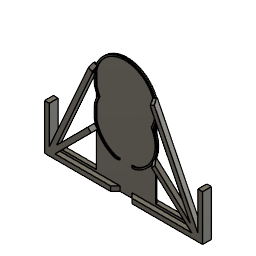
single_jig_wafer_indexer (Autodesk Fusion 360 design; units mm, degrees)
part number: 2026-08-07-17-12-09-687
Autodesk Fusion 360 part; units mm, degrees
(part 1 of 2)
ref_plane "WorkPlane1" through (0, 0, 2) normal (0, 0, 1) x (1, 0, 0)
ref_plane "WorkPlane2" through (0, 0, 3.5) normal (0, 0, 1) x (1, 0, 0)
ref_plane "WorkPlane3" through (0, 0, 10) normal (0, 0, 1) x (1, 0, 0)
ref_plane "WorkPlane4" through (0, 0, 10.2) normal (0, 0, 1) x (1, 0, 0)
ref_plane "WorkPlane5" through (0, 0, -5) normal (0, 0, 1) x (1, 0, 0)
sketch "Front Nest Base Sketch" plane through (0, 0, 0) normal (0, 0, 1) x (1, 0, 0)
  line L0 (174.19, 84.35) -> (174.1396, 86.6618)
  line L1 (174.1396, 86.6618) -> (173.9883, 88.9693)
  line L2 (173.9883, 88.9693) -> (173.7366, 91.2679)
  line L3 (173.7366, 91.2679) -> (173.3848, 93.5534)
  line L4 (173.3848, 93.5534) -> (172.9337, 95.8213)
  line L5 (172.9337, 95.8213) -> (172.3841, 98.0674)
  line L6 (172.3841, 98.0674) -> (171.737, 100.2874)
  line L7 (171.737, 100.2874) -> (170.9937, 102.4771)
  line L8 (170.9937, 102.4771) -> (170.1556, 104.6322)
  line L9 (170.1556, 104.6322) -> (169.2243, 106.7488)
  line L10 (169.2243, 106.7488) -> (168.2016, 108.8227)
  line L11 (168.2016, 108.8227) -> (167.0893, 110.85)
  line L12 (167.0893, 110.85) -> (165.8897, 112.8269)
  line L13 (165.8897, 112.8269) -> (164.6051, 114.7496)
  line L14 (164.6051, 114.7496) -> (163.2377, 116.6144)
  line L15 (163.2377, 116.6144) -> (161.7904, 118.4177)
  line L16 (161.7904, 118.4177) -> (160.2657, 120.1563)
  line L17 (160.2657, 120.1563) -> (158.6667, 121.8267)
  line L18 (158.6667, 121.8267) -> (156.9963, 123.4257)
  line L19 (156.9963, 123.4257) -> (155.2577, 124.9504)
  line L20 (155.2577, 124.9504) -> (153.4544, 126.3977)
  line L21 (153.4544, 126.3977) -> (151.5896, 127.7651)
  line L22 (151.5896, 127.7651) -> (149.6669, 129.0497)
  line L23 (149.6669, 129.0497) -> (147.69, 130.2493)
  line L24 (147.69, 130.2493) -> (145.6627, 131.3616)
  line L25 (145.6627, 131.3616) -> (143.5888, 132.3843)
  line L26 (143.5888, 132.3843) -> (141.4722, 133.3156)
  line L27 (141.4722, 133.3156) -> (139.3171, 134.1537)
  line L28 (139.3171, 134.1537) -> (137.1274, 134.897)
  line L29 (137.1274, 134.897) -> (134.9074, 135.5441)
  line L30 (134.9074, 135.5441) -> (132.6613, 136.0937)
  line L31 (132.6613, 136.0937) -> (130.3934, 136.5448)
  line L32 (130.3934, 136.5448) -> (128.1079, 136.8966)
  line L33 (128.1079, 136.8966) -> (125.8093, 137.1483)
  line L34 (125.8093, 137.1483) -> (123.5018, 137.2996)
  line L35 (123.5018, 137.2996) -> (121.19, 137.35)
  line L36 (121.19, 137.35) -> (118.8782, 137.2996)
  line L37 (118.8782, 137.2996) -> (116.5707, 137.1483)
  line L38 (116.5707, 137.1483) -> (114.2721, 136.8966)
  line L39 (114.2721, 136.8966) -> (111.9866, 136.5448)
  line L40 (111.9866, 136.5448) -> (109.7187, 136.0937)
  line L41 (109.7187, 136.0937) -> (107.4726, 135.5441)
  line L42 (107.4726, 135.5441) -> (105.2526, 134.897)
  line L43 (105.2526, 134.897) -> (103.0629, 134.1537)
  line L44 (103.0629, 134.1537) -> (100.9078, 133.3156)
  line L45 (100.9078, 133.3156) -> (98.7912, 132.3843)
  line L46 (98.7912, 132.3843) -> (96.7173, 131.3616)
  line L47 (96.7173, 131.3616) -> (94.69, 130.2493)
  line L48 (94.69, 130.2493) -> (92.7131, 129.0497)
  line L49 (92.7131, 129.0497) -> (90.7904, 127.7651)
  line L50 (90.7904, 127.7651) -> (88.9256, 126.3977)
  line L51 (88.9256, 126.3977) -> (87.1223, 124.9504)
  line L52 (87.1223, 124.9504) -> (85.3837, 123.4257)
  line L53 (85.3837, 123.4257) -> (83.7133, 121.8267)
  line L54 (83.7133, 121.8267) -> (82.1143, 120.1563)
  line L55 (82.1143, 120.1563) -> (80.5896, 118.4177)
  line L56 (80.5896, 118.4177) -> (79.1423, 116.6144)
  line L57 (79.1423, 116.6144) -> (77.7749, 114.7496)
  line L58 (77.7749, 114.7496) -> (76.4903, 112.8269)
  line L59 (76.4903, 112.8269) -> (75.2907, 110.85)
  line L60 (75.2907, 110.85) -> (74.1784, 108.8227)
  line L61 (74.1784, 108.8227) -> (73.1557, 106.7488)
  line L62 (73.1557, 106.7488) -> (72.2244, 104.6322)
  line L63 (72.2244, 104.6322) -> (71.3863, 102.4771)
  line L64 (71.3863, 102.4771) -> (70.643, 100.2874)
  line L65 (70.643, 100.2874) -> (69.9959, 98.0674)
  line L66 (69.9959, 98.0674) -> (69.4463, 95.8213)
  line L67 (69.4463, 95.8213) -> (69.0067, 93.6111)
  line L68 (69.0067, 93.6111) -> (69.0067, 75.0889)
  line L69 (69.0067, 75.0889) -> (69.4463, 72.8787)
  line L70 (69.4463, 72.8787) -> (69.9959, 70.6326)
  line L71 (69.9959, 70.6326) -> (70.643, 68.4126)
  line L72 (70.643, 68.4126) -> (71.3863, 66.2229)
  line L73 (71.3863, 66.2229) -> (72.2244, 64.0678)
  line L74 (72.2244, 64.0678) -> (73.1557, 61.9512)
  line L75 (73.1557, 61.9512) -> (74.1784, 59.8773)
  line L76 (74.1784, 59.8773) -> (75.2907, 57.85)
  line L77 (75.2907, 57.85) -> (76.4903, 55.8731)
  line L78 (76.4903, 55.8731) -> (77.7749, 53.9504)
  line L79 (77.7749, 53.9504) -> (79.1423, 52.0856)
  line L80 (79.1423, 52.0856) -> (80.5896, 50.2823)
  line L81 (80.5896, 50.2823) -> (82.1143, 48.5437)
  line L82 (82.1143, 48.5437) -> (83.7133, 46.8733)
  line L83 (83.7133, 46.8733) -> (85.3837, 45.2743)
  line L84 (85.3837, 45.2743) -> (87.1223, 43.7496)
  line L85 (87.1223, 43.7496) -> (88.9256, 42.3023)
  line L86 (88.9256, 42.3023) -> (90.7904, 40.9349)
  line L87 (90.7904, 40.9349) -> (92.7131, 39.6503)
  line L88 (92.7131, 39.6503) -> (94.69, 38.4507)
  line L89 (94.69, 38.4507) -> (96.7173, 37.3384)
  line L90 (96.7173, 37.3384) -> (98.7912, 36.3157)
  line L91 (98.7912, 36.3157) -> (100.9078, 35.3844)
  line L92 (100.9078, 35.3844) -> (103.0629, 34.5463)
  line L93 (103.0629, 34.5463) -> (104.4828, 34.0643)
  line L94 (104.4828, 34.0643) -> (137.8972, 34.0643)
  line L95 (137.8972, 34.0643) -> (139.3171, 34.5463)
  line L96 (139.3171, 34.5463) -> (141.4722, 35.3844)
  line L97 (141.4722, 35.3844) -> (143.5888, 36.3157)
  line L98 (143.5888, 36.3157) -> (145.6627, 37.3384)
  line L99 (145.6627, 37.3384) -> (147.69, 38.4507)
  line L100 (147.69, 38.4507) -> (149.6669, 39.6503)
  line L101 (149.6669, 39.6503) -> (151.5896, 40.9349)
  line L102 (151.5896, 40.9349) -> (153.4544, 42.3023)
  line L103 (153.4544, 42.3023) -> (155.2577, 43.7496)
  line L104 (155.2577, 43.7496) -> (156.9963, 45.2743)
  line L105 (156.9963, 45.2743) -> (158.6667, 46.8733)
  line L106 (158.6667, 46.8733) -> (160.2657, 48.5437)
  line L107 (160.2657, 48.5437) -> (161.7904, 50.2823)
  line L108 (161.7904, 50.2823) -> (163.2377, 52.0856)
  line L109 (163.2377, 52.0856) -> (164.6051, 53.9504)
  line L110 (164.6051, 53.9504) -> (165.8897, 55.8731)
  line L111 (165.8897, 55.8731) -> (167.0893, 57.85)
  line L112 (167.0893, 57.85) -> (168.2016, 59.8773)
  line L113 (168.2016, 59.8773) -> (169.2243, 61.9512)
  line L114 (169.2243, 61.9512) -> (170.1556, 64.0678)
  line L115 (170.1556, 64.0678) -> (170.9937, 66.2229)
  line L116 (170.9937, 66.2229) -> (171.737, 68.4126)
  line L117 (171.737, 68.4126) -> (172.3841, 70.6326)
  line L118 (172.3841, 70.6326) -> (172.9337, 72.8787)
  line L119 (172.9337, 72.8787) -> (173.3848, 75.1466)
  line L120 (173.3848, 75.1466) -> (173.7366, 77.4321)
  line L121 (173.7366, 77.4321) -> (173.9883, 79.7307)
  line L122 (173.9883, 79.7307) -> (174.1396, 82.0382)
  line L123 (174.1396, 82.0382) -> (174.19, 84.35)
extrude "Front Nest Base" add sketch "Front Nest Base Sketch" along normal blind 2
sketch "Rear Nest Base Sketch" plane through (0, 0, 0) normal (0, 0, 1) x (1, 0, 0)
  line L0 (174.19, 134.35) -> (174.1396, 136.6618)
  line L1 (174.1396, 136.6618) -> (173.9883, 138.9693)
  line L2 (173.9883, 138.9693) -> (173.7366, 141.2679)
  line L3 (173.7366, 141.2679) -> (173.3848, 143.5534)
  line L4 (173.3848, 143.5534) -> (172.9337, 145.8213)
  line L5 (172.9337, 145.8213) -> (172.3841, 148.0674)
  line L6 (172.3841, 148.0674) -> (171.737, 150.2874)
  line L7 (171.737, 150.2874) -> (170.9937, 152.4771)
  line L8 (170.9937, 152.4771) -> (170.1556, 154.6322)
  line L9 (170.1556, 154.6322) -> (169.2243, 156.7488)
  line L10 (169.2243, 156.7488) -> (168.2016, 158.8227)
  line L11 (168.2016, 158.8227) -> (167.0893, 160.85)
  line L12 (167.0893, 160.85) -> (165.8897, 162.8269)
  line L13 (165.8897, 162.8269) -> (164.6051, 164.7496)
  line L14 (164.6051, 164.7496) -> (163.2377, 166.6144)
  line L15 (163.2377, 166.6144) -> (161.7904, 168.4177)
  line L16 (161.7904, 168.4177) -> (160.2657, 170.1563)
  line L17 (160.2657, 170.1563) -> (158.6667, 171.8267)
  line L18 (158.6667, 171.8267) -> (156.9963, 173.4257)
  line L19 (156.9963, 173.4257) -> (155.2577, 174.9504)
  line L20 (155.2577, 174.9504) -> (153.4544, 176.3977)
  line L21 (153.4544, 176.3977) -> (151.5896, 177.7651)
  line L22 (151.5896, 177.7651) -> (149.6669, 179.0497)
  line L23 (149.6669, 179.0497) -> (147.69, 180.2493)
  line L24 (147.69, 180.2493) -> (145.6627, 181.3616)
  line L25 (145.6627, 181.3616) -> (143.5888, 182.3843)
  line L26 (143.5888, 182.3843) -> (141.4722, 183.3156)
  line L27 (141.4722, 183.3156) -> (139.3171, 184.1537)
  line L28 (139.3171, 184.1537) -> (137.1274, 184.897)
  line L29 (137.1274, 184.897) -> (134.9074, 185.5441)
  line L30 (134.9074, 185.5441) -> (132.6613, 186.0937)
  line L31 (132.6613, 186.0937) -> (130.3934, 186.5448)
  line L32 (130.3934, 186.5448) -> (128.1079, 186.8966)
  line L33 (128.1079, 186.8966) -> (125.8093, 187.1483)
  line L34 (125.8093, 187.1483) -> (123.5018, 187.2996)
  line L35 (123.5018, 187.2996) -> (121.19, 187.35)
  line L36 (121.19, 187.35) -> (118.8782, 187.2996)
  line L37 (118.8782, 187.2996) -> (116.5707, 187.1483)
  line L38 (116.5707, 187.1483) -> (114.2721, 186.8966)
  line L39 (114.2721, 186.8966) -> (111.9866, 186.5448)
  line L40 (111.9866, 186.5448) -> (109.7187, 186.0937)
  line L41 (109.7187, 186.0937) -> (107.4726, 185.5441)
  line L42 (107.4726, 185.5441) -> (105.2526, 184.897)
  line L43 (105.2526, 184.897) -> (103.0629, 184.1537)
  line L44 (103.0629, 184.1537) -> (100.9078, 183.3156)
  line L45 (100.9078, 183.3156) -> (98.7912, 182.3843)
  line L46 (98.7912, 182.3843) -> (96.7173, 181.3616)
  line L47 (96.7173, 181.3616) -> (94.69, 180.2493)
  line L48 (94.69, 180.2493) -> (92.7131, 179.0497)
  line L49 (92.7131, 179.0497) -> (90.7904, 177.7651)
  line L50 (90.7904, 177.7651) -> (88.9256, 176.3977)
  line L51 (88.9256, 176.3977) -> (87.1223, 174.9504)
  line L52 (87.1223, 174.9504) -> (85.3837, 173.4257)
  line L53 (85.3837, 173.4257) -> (83.7133, 171.8267)
  line L54 (83.7133, 171.8267) -> (82.1143, 170.1563)
  line L55 (82.1143, 170.1563) -> (80.5896, 168.4177)
  line L56 (80.5896, 168.4177) -> (79.1423, 166.6144)
  line L57 (79.1423, 166.6144) -> (77.7749, 164.7496)
  line L58 (77.7749, 164.7496) -> (76.4903, 162.8269)
  line L59 (76.4903, 162.8269) -> (75.2907, 160.85)
  line L60 (75.2907, 160.85) -> (74.1784, 158.8227)
  line L61 (74.1784, 158.8227) -> (73.1557, 156.7488)
  line L62 (73.1557, 156.7488) -> (72.2244, 154.6322)
  line L63 (72.2244, 154.6322) -> (71.3863, 152.4771)
  line L64 (71.3863, 152.4771) -> (70.643, 150.2874)
  line L65 (70.643, 150.2874) -> (69.9959, 148.0674)
  line L66 (69.9959, 148.0674) -> (69.4463, 145.8213)
  line L67 (69.4463, 145.8213) -> (69.0067, 143.6111)
  line L68 (69.0067, 143.6111) -> (69.0067, 125.0889)
  line L69 (69.0067, 125.0889) -> (69.4463, 122.8787)
  line L70 (69.4463, 122.8787) -> (69.9959, 120.6326)
  line L71 (69.9959, 120.6326) -> (70.643, 118.4126)
  line L72 (70.643, 118.4126) -> (71.3863, 116.2229)
  line L73 (71.3863, 116.2229) -> (72.2244, 114.0678)
  line L74 (72.2244, 114.0678) -> (73.1557, 111.9512)
  line L75 (73.1557, 111.9512) -> (74.1784, 109.8773)
  line L76 (74.1784, 109.8773) -> (75.2907, 107.85)
  line L77 (75.2907, 107.85) -> (76.4903, 105.8731)
  line L78 (76.4903, 105.8731) -> (77.7749, 103.9504)
  line L79 (77.7749, 103.9504) -> (79.1423, 102.0856)
  line L80 (79.1423, 102.0856) -> (80.5896, 100.2823)
  line L81 (80.5896, 100.2823) -> (82.1143, 98.5437)
  line L82 (82.1143, 98.5437) -> (83.7133, 96.8733)
  line L83 (83.7133, 96.8733) -> (85.3837, 95.2743)
  line L84 (85.3837, 95.2743) -> (87.1223, 93.7496)
  line L85 (87.1223, 93.7496) -> (88.9256, 92.3023)
  line L86 (88.9256, 92.3023) -> (90.7904, 90.9349)
  line L87 (90.7904, 90.9349) -> (92.7131, 89.6503)
  line L88 (92.7131, 89.6503) -> (94.69, 88.4507)
  line L89 (94.69, 88.4507) -> (96.7173, 87.3384)
  line L90 (96.7173, 87.3384) -> (98.7912, 86.3157)
  line L91 (98.7912, 86.3157) -> (100.9078, 85.3844)
  line L92 (100.9078, 85.3844) -> (103.0629, 84.5463)
  line L93 (103.0629, 84.5463) -> (104.4828, 84.0643)
  line L94 (104.4828, 84.0643) -> (137.8972, 84.0643)
  line L95 (137.8972, 84.0643) -> (139.3171, 84.5463)
  line L96 (139.3171, 84.5463) -> (141.4722, 85.3844)
  line L97 (141.4722, 85.3844) -> (143.5888, 86.3157)
  line L98 (143.5888, 86.3157) -> (145.6627, 87.3384)
  line L99 (145.6627, 87.3384) -> (147.69, 88.4507)
  line L100 (147.69, 88.4507) -> (149.6669, 89.6503)
  line L101 (149.6669, 89.6503) -> (151.5896, 90.9349)
  line L102 (151.5896, 90.9349) -> (153.4544, 92.3023)
  line L103 (153.4544, 92.3023) -> (155.2577, 93.7496)
  line L104 (155.2577, 93.7496) -> (156.9963, 95.2743)
  line L105 (156.9963, 95.2743) -> (158.6667, 96.8733)
  line L106 (158.6667, 96.8733) -> (160.2657, 98.5437)
  line L107 (160.2657, 98.5437) -> (161.7904, 100.2823)
  line L108 (161.7904, 100.2823) -> (163.2377, 102.0856)
  line L109 (163.2377, 102.0856) -> (164.6051, 103.9504)
  line L110 (164.6051, 103.9504) -> (165.8897, 105.8731)
  line L111 (165.8897, 105.8731) -> (167.0893, 107.85)
  line L112 (167.0893, 107.85) -> (168.2016, 109.8773)
  line L113 (168.2016, 109.8773) -> (169.2243, 111.9512)
  line L114 (169.2243, 111.9512) -> (170.1556, 114.0678)
  line L115 (170.1556, 114.0678) -> (170.9937, 116.2229)
  line L116 (170.9937, 116.2229) -> (171.737, 118.4126)
  line L117 (171.737, 118.4126) -> (172.3841, 120.6326)
  line L118 (172.3841, 120.6326) -> (172.9337, 122.8787)
  line L119 (172.9337, 122.8787) -> (173.3848, 125.1466)
  line L120 (173.3848, 125.1466) -> (173.7366, 127.4321)
  line L121 (173.7366, 127.4321) -> (173.9883, 129.7307)
  line L122 (173.9883, 129.7307) -> (174.1396, 132.0382)
  line L123 (174.1396, 132.0382) -> (174.19, 134.35)
extrude "Rear Nest Base" add sketch "Rear Nest Base Sketch" along normal blind 2
sketch "100 mm Structural Sheet to Rear Nest Centerline Sketch" plane through (0, 0, 0) normal (0, 0, 1) x (1, 0, 0)
  line L0 (71.19, -0.5) -> (171.19, -0.5)
  line L1 (171.19, -0.5) -> (171.19, 134.35)
  line L2 (171.19, 134.35) -> (71.19, 134.35)
  line L3 (71.19, 134.35) -> (71.19, -0.5)
extrude "100 mm Structural Sheet to Rear Nest Centerline" add sketch "100 mm Structural Sheet to Rear Nest Centerline Sketch" along normal blind 2
sketch "Front Outer Wall Sketch" plane through (0, 0, 2) normal (0, 0, 1) x (1, 0, 0)
  line L0 (174.19, 84.35) -> (174.1396, 86.6618)
  line L1 (174.1396, 86.6618) -> (173.9883, 88.9693)
  line L2 (173.9883, 88.9693) -> (173.7366, 91.2679)
  line L3 (173.7366, 91.2679) -> (173.3848, 93.5534)
  line L4 (173.3848, 93.5534) -> (172.9337, 95.8213)
  line L5 (172.9337, 95.8213) -> (172.3841, 98.0674)
  line L6 (172.3841, 98.0674) -> (171.737, 100.2874)
  line L7 (171.737, 100.2874) -> (170.9937, 102.4771)
  line L8 (170.9937, 102.4771) -> (170.1556, 104.6322)
  line L9 (170.1556, 104.6322) -> (169.2243, 106.7488)
  line L10 (169.2243, 106.7488) -> (168.2016, 108.8227)
  line L11 (168.2016, 108.8227) -> (167.0893, 110.85)
  line L12 (167.0893, 110.85) -> (165.8897, 112.8269)
  line L13 (165.8897, 112.8269) -> (164.6051, 114.7496)
  line L14 (164.6051, 114.7496) -> (163.2377, 116.6144)
  line L15 (163.2377, 116.6144) -> (161.7904, 118.4177)
  line L16 (161.7904, 118.4177) -> (160.2657, 120.1563)
  line L17 (160.2657, 120.1563) -> (158.6667, 121.8267)
  line L18 (158.6667, 121.8267) -> (156.9963, 123.4257)
  line L19 (156.9963, 123.4257) -> (155.2577, 124.9504)
  line L20 (155.2577, 124.9504) -> (153.4544, 126.3977)
  line L21 (153.4544, 126.3977) -> (151.5896, 127.7651)
  line L22 (151.5896, 127.7651) -> (149.6669, 129.0497)
  line L23 (149.6669, 129.0497) -> (147.69, 130.2493)
  line L24 (147.69, 130.2493) -> (145.6627, 131.3616)
  line L25 (145.6627, 131.3616) -> (143.5888, 132.3843)
  line L26 (143.5888, 132.3843) -> (141.4722, 133.3156)
  line L27 (141.4722, 133.3156) -> (139.3171, 134.1537)
  line L28 (139.3171, 134.1537) -> (137.1274, 134.897)
  line L29 (137.1274, 134.897) -> (134.9074, 135.5441)
  line L30 (134.9074, 135.5441) -> (132.6613, 136.0937)
  line L31 (132.6613, 136.0937) -> (130.3934, 136.5448)
  line L32 (130.3934, 136.5448) -> (128.1079, 136.8966)
  line L33 (128.1079, 136.8966) -> (125.8093, 137.1483)
  line L34 (125.8093, 137.1483) -> (123.5018, 137.2996)
  line L35 (123.5018, 137.2996) -> (121.19, 137.35)
  line L36 (121.19, 137.35) -> (118.8782, 137.2996)
  line L37 (118.8782, 137.2996) -> (116.5707, 137.1483)
  line L38 (116.5707, 137.1483) -> (114.2721, 136.8966)
  line L39 (114.2721, 136.8966) -> (111.9866, 136.5448)
  line L40 (111.9866, 136.5448) -> (109.7187, 136.0937)
  line L41 (109.7187, 136.0937) -> (107.4726, 135.5441)
  line L42 (107.4726, 135.5441) -> (105.2526, 134.897)
  line L43 (105.2526, 134.897) -> (103.0629, 134.1537)
  line L44 (103.0629, 134.1537) -> (100.9078, 133.3156)
  line L45 (100.9078, 133.3156) -> (98.7912, 132.3843)
  line L46 (98.7912, 132.3843) -> (96.7173, 131.3616)
  line L47 (96.7173, 131.3616) -> (94.69, 130.2493)
  line L48 (94.69, 130.2493) -> (92.7131, 129.0497)
  line L49 (92.7131, 129.0497) -> (90.7904, 127.7651)
  line L50 (90.7904, 127.7651) -> (88.9256, 126.3977)
  line L51 (88.9256, 126.3977) -> (87.1223, 124.9504)
  line L52 (87.1223, 124.9504) -> (85.3837, 123.4257)
  line L53 (85.3837, 123.4257) -> (83.7133, 121.8267)
  line L54 (83.7133, 121.8267) -> (82.1143, 120.1563)
  line L55 (82.1143, 120.1563) -> (80.5896, 118.4177)
  line L56 (80.5896, 118.4177) -> (79.1423, 116.6144)
  line L57 (79.1423, 116.6144) -> (77.7749, 114.7496)
  line L58 (77.7749, 114.7496) -> (76.4903, 112.8269)
  line L59 (76.4903, 112.8269) -> (75.2907, 110.85)
  line L60 (75.2907, 110.85) -> (74.1784, 108.8227)
  line L61 (74.1784, 108.8227) -> (73.1557, 106.7488)
  line L62 (73.1557, 106.7488) -> (72.2244, 104.6322)
  line L63 (72.2244, 104.6322) -> (71.3863, 102.4771)
  line L64 (71.3863, 102.4771) -> (70.643, 100.2874)
  line L65 (70.643, 100.2874) -> (69.9959, 98.0674)
  line L66 (69.9959, 98.0674) -> (69.4463, 95.8213)
  line L67 (69.4463, 95.8213) -> (69.0067, 93.6111)
  line L68 (69.0067, 93.6111) -> (69.0067, 75.0889)
  line L69 (69.0067, 75.0889) -> (69.4463, 72.8787)
  line L70 (69.4463, 72.8787) -> (69.9959, 70.6326)
  line L71 (69.9959, 70.6326) -> (70.643, 68.4126)
  line L72 (70.643, 68.4126) -> (71.3863, 66.2229)
  line L73 (71.3863, 66.2229) -> (72.2244, 64.0678)
  line L74 (72.2244, 64.0678) -> (73.1557, 61.9512)
  line L75 (73.1557, 61.9512) -> (74.1784, 59.8773)
  line L76 (74.1784, 59.8773) -> (75.2907, 57.85)
  line L77 (75.2907, 57.85) -> (76.4903, 55.8731)
  line L78 (76.4903, 55.8731) -> (77.7749, 53.9504)
  line L79 (77.7749, 53.9504) -> (79.1423, 52.0856)
  line L80 (79.1423, 52.0856) -> (80.5896, 50.2823)
  line L81 (80.5896, 50.2823) -> (82.1143, 48.5437)
  line L82 (82.1143, 48.5437) -> (83.7133, 46.8733)
  line L83 (83.7133, 46.8733) -> (85.3837, 45.2743)
  line L84 (85.3837, 45.2743) -> (87.1223, 43.7496)
  line L85 (87.1223, 43.7496) -> (88.9256, 42.3023)
  line L86 (88.9256, 42.3023) -> (90.7904, 40.9349)
  line L87 (90.7904, 40.9349) -> (92.7131, 39.6503)
  line L88 (92.7131, 39.6503) -> (94.69, 38.4507)
  line L89 (94.69, 38.4507) -> (96.7173, 37.3384)
  line L90 (96.7173, 37.3384) -> (98.7912, 36.3157)
  line L91 (98.7912, 36.3157) -> (100.9078, 35.3844)
  line L92 (100.9078, 35.3844) -> (103.0629, 34.5463)
  line L93 (103.0629, 34.5463) -> (104.4828, 34.0643)
  line L94 (104.4828, 34.0643) -> (137.8972, 34.0643)
  line L95 (137.8972, 34.0643) -> (139.3171, 34.5463)
  line L96 (139.3171, 34.5463) -> (141.4722, 35.3844)
  line L97 (141.4722, 35.3844) -> (143.5888, 36.3157)
  line L98 (143.5888, 36.3157) -> (145.6627, 37.3384)
  line L99 (145.6627, 37.3384) -> (147.69, 38.4507)
  line L100 (147.69, 38.4507) -> (149.6669, 39.6503)
  line L101 (149.6669, 39.6503) -> (151.5896, 40.9349)
  line L102 (151.5896, 40.9349) -> (153.4544, 42.3023)
  line L103 (153.4544, 42.3023) -> (155.2577, 43.7496)
  line L104 (155.2577, 43.7496) -> (156.9963, 45.2743)
  line L105 (156.9963, 45.2743) -> (158.6667, 46.8733)
  line L106 (158.6667, 46.8733) -> (160.2657, 48.5437)
  line L107 (160.2657, 48.5437) -> (161.7904, 50.2823)
  line L108 (161.7904, 50.2823) -> (163.2377, 52.0856)
  line L109 (163.2377, 52.0856) -> (164.6051, 53.9504)
  line L110 (164.6051, 53.9504) -> (165.8897, 55.8731)
  line L111 (165.8897, 55.8731) -> (167.0893, 57.85)
  line L112 (167.0893, 57.85) -> (168.2016, 59.8773)
  line L113 (168.2016, 59.8773) -> (169.2243, 61.9512)
  line L114 (169.2243, 61.9512) -> (170.1556, 64.0678)
  line L115 (170.1556, 64.0678) -> (170.9937, 66.2229)
  line L116 (170.9937, 66.2229) -> (171.737, 68.4126)
  line L117 (171.737, 68.4126) -> (172.3841, 70.6326)
  line L118 (172.3841, 70.6326) -> (172.9337, 72.8787)
  line L119 (172.9337, 72.8787) -> (173.3848, 75.1466)
  line L120 (173.3848, 75.1466) -> (173.7366, 77.4321)
  line L121 (173.7366, 77.4321) -> (173.9883, 79.7307)
  line L122 (173.9883, 79.7307) -> (174.1396, 82.0382)
  line L123 (174.1396, 82.0382) -> (174.19, 84.35)
extrude "Front Outer Wall" add sketch "Front Outer Wall Sketch" along normal blind 1.5
sketch "Rear Outer Wall Sketch" plane through (0, 0, 2) normal (0, 0, 1) x (1, 0, 0)
  line L0 (174.19, 134.35) -> (174.1396, 136.6618)
  line L1 (174.1396, 136.6618) -> (173.9883, 138.9693)
  line L2 (173.9883, 138.9693) -> (173.7366, 141.2679)
  line L3 (173.7366, 141.2679) -> (173.3848, 143.5534)
  line L4 (173.3848, 143.5534) -> (172.9337, 145.8213)
  line L5 (172.9337, 145.8213) -> (172.3841, 148.0674)
  line L6 (172.3841, 148.0674) -> (171.737, 150.2874)
  line L7 (171.737, 150.2874) -> (170.9937, 152.4771)
  line L8 (170.9937, 152.4771) -> (170.1556, 154.6322)
  line L9 (170.1556, 154.6322) -> (169.2243, 156.7488)
  line L10 (169.2243, 156.7488) -> (168.2016, 158.8227)
  line L11 (168.2016, 158.8227) -> (167.0893, 160.85)
  line L12 (167.0893, 160.85) -> (165.8897, 162.8269)
  line L13 (165.8897, 162.8269) -> (164.6051, 164.7496)
  line L14 (164.6051, 164.7496) -> (163.2377, 166.6144)
  line L15 (163.2377, 166.6144) -> (161.7904, 168.4177)
  line L16 (161.7904, 168.4177) -> (160.2657, 170.1563)
  line L17 (160.2657, 170.1563) -> (158.6667, 171.8267)
  line L18 (158.6667, 171.8267) -> (156.9963, 173.4257)
  line L19 (156.9963, 173.4257) -> (155.2577, 174.9504)
  line L20 (155.2577, 174.9504) -> (153.4544, 176.3977)
  line L21 (153.4544, 176.3977) -> (151.5896, 177.7651)
  line L22 (151.5896, 177.7651) -> (149.6669, 179.0497)
  line L23 (149.6669, 179.0497) -> (147.69, 180.2493)
  line L24 (147.69, 180.2493) -> (145.6627, 181.3616)
  line L25 (145.6627, 181.3616) -> (143.5888, 182.3843)
  line L26 (143.5888, 182.3843) -> (141.4722, 183.3156)
  line L27 (141.4722, 183.3156) -> (139.3171, 184.1537)
  line L28 (139.3171, 184.1537) -> (137.1274, 184.897)
  line L29 (137.1274, 184.897) -> (134.9074, 185.5441)
  line L30 (134.9074, 185.5441) -> (132.6613, 186.0937)
  line L31 (132.6613, 186.0937) -> (130.3934, 186.5448)
  line L32 (130.3934, 186.5448) -> (128.1079, 186.8966)
  line L33 (128.1079, 186.8966) -> (125.8093, 187.1483)
  line L34 (125.8093, 187.1483) -> (123.5018, 187.2996)
  line L35 (123.5018, 187.2996) -> (121.19, 187.35)
  line L36 (121.19, 187.35) -> (118.8782, 187.2996)
  line L37 (118.8782, 187.2996) -> (116.5707, 187.1483)
  line L38 (116.5707, 187.1483) -> (114.2721, 186.8966)
  line L39 (114.2721, 186.8966) -> (111.9866, 186.5448)
  line L40 (111.9866, 186.5448) -> (109.7187, 186.0937)
  line L41 (109.7187, 186.0937) -> (107.4726, 185.5441)
  line L42 (107.4726, 185.5441) -> (105.2526, 184.897)
  line L43 (105.2526, 184.897) -> (103.0629, 184.1537)
  line L44 (103.0629, 184.1537) -> (100.9078, 183.3156)
  line L45 (100.9078, 183.3156) -> (98.7912, 182.3843)
  line L46 (98.7912, 182.3843) -> (96.7173, 181.3616)
  line L47 (96.7173, 181.3616) -> (94.69, 180.2493)
  line L48 (94.69, 180.2493) -> (92.7131, 179.0497)
  line L49 (92.7131, 179.0497) -> (90.7904, 177.7651)
  line L50 (90.7904, 177.7651) -> (88.9256, 176.3977)
  line L51 (88.9256, 176.3977) -> (87.1223, 174.9504)
  line L52 (87.1223, 174.9504) -> (85.3837, 173.4257)
  line L53 (85.3837, 173.4257) -> (83.7133, 171.8267)
  line L54 (83.7133, 171.8267) -> (82.1143, 170.1563)
  line L55 (82.1143, 170.1563) -> (80.5896, 168.4177)
  line L56 (80.5896, 168.4177) -> (79.1423, 166.6144)
  line L57 (79.1423, 166.6144) -> (77.7749, 164.7496)
  line L58 (77.7749, 164.7496) -> (76.4903, 162.8269)
  line L59 (76.4903, 162.8269) -> (75.2907, 160.85)
  line L60 (75.2907, 160.85) -> (74.1784, 158.8227)
  line L61 (74.1784, 158.8227) -> (73.1557, 156.7488)
  line L62 (73.1557, 156.7488) -> (72.2244, 154.6322)
  line L63 (72.2244, 154.6322) -> (71.3863, 152.4771)
  line L64 (71.3863, 152.4771) -> (70.643, 150.2874)
  line L65 (70.643, 150.2874) -> (69.9959, 148.0674)
  line L66 (69.9959, 148.0674) -> (69.4463, 145.8213)
  line L67 (69.4463, 145.8213) -> (69.0067, 143.6111)
  line L68 (69.0067, 143.6111) -> (69.0067, 125.0889)
  line L69 (69.0067, 125.0889) -> (69.4463, 122.8787)
  line L70 (69.4463, 122.8787) -> (69.9959, 120.6326)
  line L71 (69.9959, 120.6326) -> (70.643, 118.4126)
  line L72 (70.643, 118.4126) -> (71.3863, 116.2229)
  line L73 (71.3863, 116.2229) -> (72.2244, 114.0678)
  line L74 (72.2244, 114.0678) -> (73.1557, 111.9512)
  line L75 (73.1557, 111.9512) -> (74.1784, 109.8773)
  line L76 (74.1784, 109.8773) -> (75.2907, 107.85)
  line L77 (75.2907, 107.85) -> (76.4903, 105.8731)
  line L78 (76.4903, 105.8731) -> (77.7749, 103.9504)
  line L79 (77.7749, 103.9504) -> (79.1423, 102.0856)
  line L80 (79.1423, 102.0856) -> (80.5896, 100.2823)
  line L81 (80.5896, 100.2823) -> (82.1143, 98.5437)
  line L82 (82.1143, 98.5437) -> (83.7133, 96.8733)
  line L83 (83.7133, 96.8733) -> (85.3837, 95.2743)
  line L84 (85.3837, 95.2743) -> (87.1223, 93.7496)
  line L85 (87.1223, 93.7496) -> (88.9256, 92.3023)
  line L86 (88.9256, 92.3023) -> (90.7904, 90.9349)
  line L87 (90.7904, 90.9349) -> (92.7131, 89.6503)
  line L88 (92.7131, 89.6503) -> (94.69, 88.4507)
  line L89 (94.69, 88.4507) -> (96.7173, 87.3384)
  line L90 (96.7173, 87.3384) -> (98.7912, 86.3157)
  line L91 (98.7912, 86.3157) -> (100.9078, 85.3844)
  line L92 (100.9078, 85.3844) -> (103.0629, 84.5463)
  line L93 (103.0629, 84.5463) -> (104.4828, 84.0643)
  line L94 (104.4828, 84.0643) -> (137.8972, 84.0643)
  line L95 (137.8972, 84.0643) -> (139.3171, 84.5463)
  line L96 (139.3171, 84.5463) -> (141.4722, 85.3844)
  line L97 (141.4722, 85.3844) -> (143.5888, 86.3157)
  line L98 (143.5888, 86.3157) -> (145.6627, 87.3384)
  line L99 (145.6627, 87.3384) -> (147.69, 88.4507)
  line L100 (147.69, 88.4507) -> (149.6669, 89.6503)
  line L101 (149.6669, 89.6503) -> (151.5896, 90.9349)
  line L102 (151.5896, 90.9349) -> (153.4544, 92.3023)
  line L103 (153.4544, 92.3023) -> (155.2577, 93.7496)
  line L104 (155.2577, 93.7496) -> (156.9963, 95.2743)
  line L105 (156.9963, 95.2743) -> (158.6667, 96.8733)
  line L106 (158.6667, 96.8733) -> (160.2657, 98.5437)
  line L107 (160.2657, 98.5437) -> (161.7904, 100.2823)
  line L108 (161.7904, 100.2823) -> (163.2377, 102.0856)
  line L109 (163.2377, 102.0856) -> (164.6051, 103.9504)
  line L110 (164.6051, 103.9504) -> (165.8897, 105.8731)
  line L111 (165.8897, 105.8731) -> (167.0893, 107.85)
  line L112 (167.0893, 107.85) -> (168.2016, 109.8773)
  line L113 (168.2016, 109.8773) -> (169.2243, 111.9512)
  line L114 (169.2243, 111.9512) -> (170.1556, 114.0678)
  line L115 (170.1556, 114.0678) -> (170.9937, 116.2229)
  line L116 (170.9937, 116.2229) -> (171.737, 118.4126)
  line L117 (171.737, 118.4126) -> (172.3841, 120.6326)
  line L118 (172.3841, 120.6326) -> (172.9337, 122.8787)
  line L119 (172.9337, 122.8787) -> (173.3848, 125.1466)
  line L120 (173.3848, 125.1466) -> (173.7366, 127.4321)
  line L121 (173.7366, 127.4321) -> (173.9883, 129.7307)
  line L122 (173.9883, 129.7307) -> (174.1396, 132.0382)
  line L123 (174.1396, 132.0382) -> (174.19, 134.35)
extrude "Rear Outer Wall" add sketch "Rear Outer Wall Sketch" along normal blind 1.5
sketch "Front Table Bar Sketch" plane through (0, 0, -5) normal (0, 0, 1) x (1, 0, 0)
  line L0 (-8, -12) -> (258, -12)
  line L1 (258, -12) -> (258, 0)
  line L2 (258, 0) -> (-8, 0)
  line L3 (-8, 0) -> (-8, -12)
extrude "Front Table Bar" add sketch "Front Table Bar Sketch" along normal blind 7
sketch "Left Table Bar Sketch" plane through (0, 0, -5) normal (0, 0, 1) x (1, 0, 0)
  line L0 (-8, -12) -> (0, -12)
  line L1 (0, -12) -> (0, 65)
  line L2 (0, 65) -> (-8, 65)
  line L3 (-8, 65) -> (-8, -12)
extrude "Left Table Bar" add sketch "Left Table Bar Sketch" along normal blind 15
sketch "Right Table Bar Sketch" plane through (0, 0, -5) normal (0, 0, 1) x (1, 0, 0)
  line L0 (250, -12) -> (258, -12)
  line L1 (258, -12) -> (258, 65)
  line L2 (258, 65) -> (250, 65)
  line L3 (250, 65) -> (250, -12)
extrude "Right Table Bar" add sketch "Right Table Bar Sketch" along normal blind 15
sketch "Continuous Front Top Rib Sketch" plane through (0, 0, 2) normal (0, 0, 1) x (1, 0, 0)
  line L0 (-8, -12) -> (258, -12)
  line L1 (258, -12) -> (258, -4)
  line L2 (258, -4) -> (-8, -4)
  line L3 (-8, -4) -> (-8, -12)
extrude "Continuous Front Top Rib" add sketch "Continuous Front Top Rib Sketch" along normal blind 8
sketch "Left Front Diagonal Rib Lower Web Sketch" plane through (0, 0, 2) normal (0, 0, 1) x (1, 0, 0)
  line L0 (-2.8332, -5.1763) -> (69.2753, 67.1737)
  line L1 (69.2753, 67.1737) -> (74.9416, 61.5263)
  line L2 (74.9416, 61.5263) -> (2.8332, -10.8237)
  line L3 (2.8332, -10.8237) -> (-2.8332, -5.1763)
extrude "Left Front Diagonal Rib Lower Web" add sketch "Left Front Diagonal Rib Lower Web Sketch" along normal blind 1.5
sketch "Left Front Diagonal Rib 45 Degree Thickness Taper Lower Sketch" plane through (0, 0, 3.5) normal (0, 0, 1) x (1, 0, 0)
  line L0 (-2.8332, -5.1763) -> (69.2753, 67.1737)
  line L1 (69.2753, 67.1737) -> (74.9416, 61.5263)
  line L2 (74.9416, 61.5263) -> (2.8332, -10.8237)
  line L3 (2.8332, -10.8237) -> (-2.8332, -5.1763)
sketch "Left Front Diagonal Rib 45 Degree Thickness Taper Upper Sketch" plane through (0, 0, 10) normal (0, 0, 1) x (1, 0, 0)
  line L0 (-2.8332, -5.1763) -> (64.6868, 62.5698)
  line L1 (64.6868, 62.5698) -> (70.3531, 56.9224)
  line L2 (70.3531, 56.9224) -> (2.8332, -10.8237)
  line L3 (2.8332, -10.8237) -> (-2.8332, -5.1763)
loft "Left Front Diagonal Rib 45 Degree Thickness Taper" add profiles "Left Front Diagonal Rib 45 Degree Thickness Taper Lower Sketch", "Left Front Diagonal Rib 45 Degree Thickness Taper Upper Sketch" section 1 section 2
sketch "Right Front Diagonal Rib Lower Web Sketch" plane through (0, 0, 2) normal (0, 0, 1) x (1, 0, 0)
  line L0 (247.312, -10.9622) -> (167.5835, 61.3878)
  line L1 (167.5835, 61.3878) -> (172.9596, 67.3122)
  line L2 (172.9596, 67.3122) -> (252.688, -5.0378)
  line L3 (252.688, -5.0378) -> (247.312, -10.9622)
extrude "Right Front Diagonal Rib Lower Web" add sketch "Right Front Diagonal Rib Lower Web Sketch" along normal blind 1.5
sketch "Right Front Diagonal Rib 45 Degree Thickness Taper Lower Sketch" plane through (0, 0, 3.5) normal (0, 0, 1) x (1, 0, 0)
  line L0 (247.312, -10.9622) -> (167.5835, 61.3878)
  line L1 (167.5835, 61.3878) -> (172.9596, 67.3122)
  line L2 (172.9596, 67.3122) -> (252.688, -5.0378)
  line L3 (252.688, -5.0378) -> (247.312, -10.9622)
sketch "Right Front Diagonal Rib 45 Degree Thickness Taper Upper Sketch" plane through (0, 0, 10) normal (0, 0, 1) x (1, 0, 0)
  line L0 (247.312, -10.9622) -> (172.3971, 57.0198)
  line L1 (172.3971, 57.0198) -> (177.7731, 62.9441)
  line L2 (177.7731, 62.9441) -> (252.688, -5.0378)
  line L3 (252.688, -5.0378) -> (247.312, -10.9622)
loft "Right Front Diagonal Rib 45 Degree Thickness Taper" add profiles "Right Front Diagonal Rib 45 Degree Thickness Taper Lower Sketch", "Right Front Diagonal Rib 45 Degree Thickness Taper Upper Sketch" section 1 section 2
sketch "Left Rear Diagonal Rib Lower Web Sketch" plane through (0, 0, 2) normal (0, 0, 1) x (1, 0, 0)
  line L0 (-3.6556, -6.3763) -> (68.4528, 155.9737)
  line L1 (68.4528, 155.9737) -> (75.7641, 152.7263)
  line L2 (75.7641, 152.7263) -> (3.6556, -9.6237)
  line L3 (3.6556, -9.6237) -> (-3.6556, -6.3763)
extrude "Left Rear Diagonal Rib Lower Web" add sketch "Left Rear Diagonal Rib Lower Web Sketch" along normal blind 1.5
sketch "Left Rear Diagonal Rib 45 Degree Thickness Taper Lower Sketch" plane through (0, 0, 3.5) normal (0, 0, 1) x (1, 0, 0)
  line L0 (-3.6556, -6.3763) -> (68.4528, 155.9737)
  line L1 (68.4528, 155.9737) -> (75.7641, 152.7263)
  line L2 (75.7641, 152.7263) -> (3.6556, -9.6237)
  line L3 (3.6556, -9.6237) -> (-3.6556, -6.3763)
sketch "Left Rear Diagonal Rib 45 Degree Thickness Taper Upper Sketch" plane through (0, 0, 10) normal (0, 0, 1) x (1, 0, 0)
  line L0 (-3.6556, -6.3763) -> (65.8143, 150.0333)
  line L1 (65.8143, 150.0333) -> (73.1256, 146.7859)
  line L2 (73.1256, 146.7859) -> (3.6556, -9.6237)
  line L3 (3.6556, -9.6237) -> (-3.6556, -6.3763)
loft "Left Rear Diagonal Rib 45 Degree Thickness Taper" add profiles "Left Rear Diagonal Rib 45 Degree Thickness Taper Lower Sketch", "Left Rear Diagonal Rib 45 Degree Thickness Taper Upper Sketch" section 1 section 2
sketch "Right Rear Diagonal Rib Lower Web Sketch" plane through (0, 0, 2) normal (0, 0, 1) x (1, 0, 0)
  line L0 (246.4096, -9.7632) -> (166.6812, 152.5868)
  line L1 (166.6812, 152.5868) -> (173.862, 156.1132)
  line L2 (173.862, 156.1132) -> (253.5904, -6.2368)
  line L3 (253.5904, -6.2368) -> (246.4096, -9.7632)
extrude "Right Rear Diagonal Rib Lower Web" add sketch "Right Rear Diagonal Rib Lower Web Sketch" along normal blind 1.5
sketch "Right Rear Diagonal Rib 45 Degree Thickness Taper Lower Sketch" plane through (0, 0, 3.5) normal (0, 0, 1) x (1, 0, 0)
  line L0 (246.4096, -9.7632) -> (166.6812, 152.5868)
  line L1 (166.6812, 152.5868) -> (173.862, 156.1132)
  line L2 (173.862, 156.1132) -> (253.5904, -6.2368)
  line L3 (253.5904, -6.2368) -> (246.4096, -9.7632)
sketch "Right Rear Diagonal Rib 45 Degree Thickness Taper Upper Sketch" plane through (0, 0, 10) normal (0, 0, 1) x (1, 0, 0)
  line L0 (246.4096, -9.7632) -> (169.5464, 146.7524)
  line L1 (169.5464, 146.7524) -> (176.7272, 150.2788)
  line L2 (176.7272, 150.2788) -> (253.5904, -6.2368)
  line L3 (253.5904, -6.2368) -> (246.4096, -9.7632)
loft "Right Rear Diagonal Rib 45 Degree Thickness Taper" add profiles "Right Rear Diagonal Rib 45 Degree Thickness Taper Lower Sketch", "Right Rear Diagonal Rib 45 Degree Thickness Taper Upper Sketch" section 1 section 2
sketch "Front Wafer Pocket - Final Clearance Sketch" plane through (0, 0, 2) normal (0, 0, 1) x (1, 0, 0)
  line L0 (171.69, 84.35) -> (171.6419, 86.5528)
  line L1 (171.6419, 86.5528) -> (171.4978, 88.7514)
  line L2 (171.4978, 88.7514) -> (171.258, 90.9416)
  line L3 (171.258, 90.9416) -> (170.9228, 93.1192)
  line L4 (170.9228, 93.1192) -> (170.4929, 95.2802)
  line L5 (170.4929, 95.2802) -> (169.9693, 97.4204)
  line L6 (169.9693, 97.4204) -> (169.3527, 99.5356)
  line L7 (169.3527, 99.5356) -> (168.6445, 101.622)
  line L8 (168.6445, 101.622) -> (167.8459, 103.6755)
  line L9 (167.8459, 103.6755) -> (166.9585, 105.6922)
  line L10 (166.9585, 105.6922) -> (165.984, 107.6683)
  line L11 (165.984, 107.6683) -> (164.9243, 109.6)
  line L12 (164.9243, 109.6) -> (163.7813, 111.4836)
  line L13 (163.7813, 111.4836) -> (162.5572, 113.3156)
  line L14 (162.5572, 113.3156) -> (161.2543, 115.0925)
  line L15 (161.2543, 115.0925) -> (159.8752, 116.8108)
  line L16 (159.8752, 116.8108) -> (158.4225, 118.4673)
  line L17 (158.4225, 118.4673) -> (156.8989, 120.0589)
  line L18 (156.8989, 120.0589) -> (155.3073, 121.5825)
  line L19 (155.3073, 121.5825) -> (153.6508, 123.0352)
  line L20 (153.6508, 123.0352) -> (151.9325, 124.4143)
  line L21 (151.9325, 124.4143) -> (150.1556, 125.7172)
  line L22 (150.1556, 125.7172) -> (148.3236, 126.9413)
  line L23 (148.3236, 126.9413) -> (146.44, 128.0843)
  line L24 (146.44, 128.0843) -> (144.5083, 129.144)
  line L25 (144.5083, 129.144) -> (142.5322, 130.1185)
  line L26 (142.5322, 130.1185) -> (140.5155, 131.0059)
  line L27 (140.5155, 131.0059) -> (138.462, 131.8045)
  line L28 (138.462, 131.8045) -> (136.3756, 132.5127)
  line L29 (136.3756, 132.5127) -> (134.2604, 133.1293)
  line L30 (134.2604, 133.1293) -> (132.1202, 133.6529)
  line L31 (132.1202, 133.6529) -> (129.9592, 134.0828)
  line L32 (129.9592, 134.0828) -> (127.7816, 134.418)
  line L33 (127.7816, 134.418) -> (125.5914, 134.6578)
  line L34 (125.5914, 134.6578) -> (123.3928, 134.8019)
  line L35 (123.3928, 134.8019) -> (121.19, 134.85)
  line L36 (121.19, 134.85) -> (118.9872, 134.8019)
  line L37 (118.9872, 134.8019) -> (116.7886, 134.6578)
  line L38 (116.7886, 134.6578) -> (114.5984, 134.418)
  line L39 (114.5984, 134.418) -> (112.4208, 134.0828)
  line L40 (112.4208, 134.0828) -> (110.2598, 133.6529)
  line L41 (110.2598, 133.6529) -> (108.1196, 133.1293)
  line L42 (108.1196, 133.1293) -> (106.0044, 132.5127)
  line L43 (106.0044, 132.5127) -> (103.918, 131.8045)
  line L44 (103.918, 131.8045) -> (101.8645, 131.0059)
  line L45 (101.8645, 131.0059) -> (99.8478, 130.1185)
  line L46 (99.8478, 130.1185) -> (97.8717, 129.144)
  line L47 (97.8717, 129.144) -> (95.94, 128.0843)
  line L48 (95.94, 128.0843) -> (94.0564, 126.9413)
  line L49 (94.0564, 126.9413) -> (92.2244, 125.7172)
  line L50 (92.2244, 125.7172) -> (90.4475, 124.4143)
  line L51 (90.4475, 124.4143) -> (88.7292, 123.0352)
  line L52 (88.7292, 123.0352) -> (87.0727, 121.5825)
  line L53 (87.0727, 121.5825) -> (85.4811, 120.0589)
  line L54 (85.4811, 120.0589) -> (83.9575, 118.4673)
  line L55 (83.9575, 118.4673) -> (82.5048, 116.8108)
  line L56 (82.5048, 116.8108) -> (81.1257, 115.0925)
  line L57 (81.1257, 115.0925) -> (79.8228, 113.3156)
  line L58 (79.8228, 113.3156) -> (78.5987, 111.4836)
  line L59 (78.5987, 111.4836) -> (77.4557, 109.6)
  line L60 (77.4557, 109.6) -> (76.396, 107.6683)
  line L61 (76.396, 107.6683) -> (75.4215, 105.6922)
  line L62 (75.4215, 105.6922) -> (74.5341, 103.6755)
  line L63 (74.5341, 103.6755) -> (73.7355, 101.622)
  line L64 (73.7355, 101.622) -> (73.0273, 99.5356)
  line L65 (73.0273, 99.5356) -> (72.4107, 97.4204)
  line L66 (72.4107, 97.4204) -> (71.9067, 95.3604)
  line L67 (71.9067, 95.3604) -> (71.9067, 73.3396)
  line L68 (71.9067, 73.3396) -> (72.4107, 71.2796)
  line L69 (72.4107, 71.2796) -> (73.0273, 69.1644)
  line L70 (73.0273, 69.1644) -> (73.7355, 67.078)
  line L71 (73.7355, 67.078) -> (74.5341, 65.0245)
  line L72 (74.5341, 65.0245) -> (75.4215, 63.0078)
  line L73 (75.4215, 63.0078) -> (76.396, 61.0317)
  line L74 (76.396, 61.0317) -> (77.4557, 59.1)
  line L75 (77.4557, 59.1) -> (78.5987, 57.2164)
  line L76 (78.5987, 57.2164) -> (79.8228, 55.3844)
  line L77 (79.8228, 55.3844) -> (81.1257, 53.6075)
  line L78 (81.1257, 53.6075) -> (82.5048, 51.8892)
  line L79 (82.5048, 51.8892) -> (83.9575, 50.2327)
  line L80 (83.9575, 50.2327) -> (85.4811, 48.6411)
  line L81 (85.4811, 48.6411) -> (87.0727, 47.1175)
  line L82 (87.0727, 47.1175) -> (88.7292, 45.6648)
  line L83 (88.7292, 45.6648) -> (90.4475, 44.2857)
  line L84 (90.4475, 44.2857) -> (92.2244, 42.9828)
  line L85 (92.2244, 42.9828) -> (94.0564, 41.7587)
  line L86 (94.0564, 41.7587) -> (95.94, 40.6157)
  line L87 (95.94, 40.6157) -> (97.8717, 39.556)
  line L88 (97.8717, 39.556) -> (99.8478, 38.5815)
  line L89 (99.8478, 38.5815) -> (101.8645, 37.6941)
  line L90 (101.8645, 37.6941) -> (103.918, 36.8955)
  line L91 (103.918, 36.8955) -> (104.8937, 36.5643)
  line L92 (104.8937, 36.5643) -> (137.4863, 36.5643)
  line L93 (137.4863, 36.5643) -> (138.462, 36.8955)
  line L94 (138.462, 36.8955) -> (140.5155, 37.6941)
  line L95 (140.5155, 37.6941) -> (142.5322, 38.5815)
  line L96 (142.5322, 38.5815) -> (144.5083, 39.556)
  line L97 (144.5083, 39.556) -> (146.44, 40.6157)
  line L98 (146.44, 40.6157) -> (148.3236, 41.7587)
  line L99 (148.3236, 41.7587) -> (150.1556, 42.9828)
  line L100 (150.1556, 42.9828) -> (151.9325, 44.2857)
  line L101 (151.9325, 44.2857) -> (153.6508, 45.6648)
  line L102 (153.6508, 45.6648) -> (155.3073, 47.1175)
  line L103 (155.3073, 47.1175) -> (156.8989, 48.6411)
  line L104 (156.8989, 48.6411) -> (158.4225, 50.2327)
  line L105 (158.4225, 50.2327) -> (159.8752, 51.8892)
  line L106 (159.8752, 51.8892) -> (161.2543, 53.6075)
  line L107 (161.2543, 53.6075) -> (162.5572, 55.3844)
  line L108 (162.5572, 55.3844) -> (163.7813, 57.2164)
  line L109 (163.7813, 57.2164) -> (164.9243, 59.1)
  line L110 (164.9243, 59.1) -> (165.984, 61.0317)
  line L111 (165.984, 61.0317) -> (166.9585, 63.0078)
  line L112 (166.9585, 63.0078) -> (167.8459, 65.0245)
  line L113 (167.8459, 65.0245) -> (168.6445, 67.078)
  line L114 (168.6445, 67.078) -> (169.3527, 69.1644)
  line L115 (169.3527, 69.1644) -> (169.9693, 71.2796)
  line L116 (169.9693, 71.2796) -> (170.4929, 73.4198)
  line L117 (170.4929, 73.4198) -> (170.9228, 75.5808)
  line L118 (170.9228, 75.5808) -> (171.258, 77.7584)
  line L119 (171.258, 77.7584) -> (171.4978, 79.9486)
  line L120 (171.4978, 79.9486) -> (171.6419, 82.1472)
  line L121 (171.6419, 82.1472) -> (171.69, 84.35)
extrude "Front Wafer Pocket - Final Clearance" cut sketch "Front Wafer Pocket - Final Clearance Sketch" along normal blind 8.1
sketch "Rear Wafer Pocket - Final Clearance Sketch" plane through (0, 0, 2) normal (0, 0, 1) x (1, 0, 0)
  line L0 (171.69, 134.35) -> (171.6419, 136.5528)
  line L1 (171.6419, 136.5528) -> (171.4978, 138.7514)
  line L2 (171.4978, 138.7514) -> (171.258, 140.9416)
  line L3 (171.258, 140.9416) -> (170.9228, 143.1192)
  line L4 (170.9228, 143.1192) -> (170.4929, 145.2802)
  line L5 (170.4929, 145.2802) -> (169.9693, 147.4204)
  line L6 (169.9693, 147.4204) -> (169.3527, 149.5356)
  line L7 (169.3527, 149.5356) -> (168.6445, 151.622)
  line L8 (168.6445, 151.622) -> (167.8459, 153.6755)
  line L9 (167.8459, 153.6755) -> (166.9585, 155.6922)
  line L10 (166.9585, 155.6922) -> (165.984, 157.6683)
  line L11 (165.984, 157.6683) -> (164.9243, 159.6)
  line L12 (164.9243, 159.6) -> (163.7813, 161.4836)
  line L13 (163.7813, 161.4836) -> (162.5572, 163.3156)
  line L14 (162.5572, 163.3156) -> (161.2543, 165.0925)
  line L15 (161.2543, 165.0925) -> (159.8752, 166.8108)
  line L16 (159.8752, 166.8108) -> (158.4225, 168.4673)
  line L17 (158.4225, 168.4673) -> (156.8989, 170.0589)
  line L18 (156.8989, 170.0589) -> (155.3073, 171.5825)
  line L19 (155.3073, 171.5825) -> (153.6508, 173.0352)
  line L20 (153.6508, 173.0352) -> (151.9325, 174.4143)
  line L21 (151.9325, 174.4143) -> (150.1556, 175.7172)
  line L22 (150.1556, 175.7172) -> (148.3236, 176.9413)
  line L23 (148.3236, 176.9413) -> (146.44, 178.0843)
  line L24 (146.44, 178.0843) -> (144.5083, 179.144)
  line L25 (144.5083, 179.144) -> (142.5322, 180.1185)
  line L26 (142.5322, 180.1185) -> (140.5155, 181.0059)
  line L27 (140.5155, 181.0059) -> (138.462, 181.8045)
  line L28 (138.462, 181.8045) -> (136.3756, 182.5127)
  line L29 (136.3756, 182.5127) -> (134.2604, 183.1293)
  line L30 (134.2604, 183.1293) -> (132.1202, 183.6529)
  line L31 (132.1202, 183.6529) -> (129.9592, 184.0828)
  line L32 (129.9592, 184.0828) -> (127.7816, 184.418)
  line L33 (127.7816, 184.418) -> (125.5914, 184.6578)
  line L34 (125.5914, 184.6578) -> (123.3928, 184.8019)
  line L35 (123.3928, 184.8019) -> (121.19, 184.85)
  line L36 (121.19, 184.85) -> (118.9872, 184.8019)
  line L37 (118.9872, 184.8019) -> (116.7886, 184.6578)
  line L38 (116.7886, 184.6578) -> (114.5984, 184.418)
  line L39 (114.5984, 184.418) -> (112.4208, 184.0828)
  line L40 (112.4208, 184.0828) -> (110.2598, 183.6529)
  line L41 (110.2598, 183.6529) -> (108.1196, 183.1293)
  line L42 (108.1196, 183.1293) -> (106.0044, 182.5127)
  line L43 (106.0044, 182.5127) -> (103.918, 181.8045)
  line L44 (103.918, 181.8045) -> (101.8645, 181.0059)
  line L45 (101.8645, 181.0059) -> (99.8478, 180.1185)
  line L46 (99.8478, 180.1185) -> (97.8717, 179.144)
  line L47 (97.8717, 179.144) -> (95.94, 178.0843)
  line L48 (95.94, 178.0843) -> (94.0564, 176.9413)
  line L49 (94.0564, 176.9413) -> (92.2244, 175.7172)
  line L50 (92.2244, 175.7172) -> (90.4475, 174.4143)
  line L51 (90.4475, 174.4143) -> (88.7292, 173.0352)
  line L52 (88.7292, 173.0352) -> (87.0727, 171.5825)
  line L53 (87.0727, 171.5825) -> (85.4811, 170.0589)
  line L54 (85.4811, 170.0589) -> (83.9575, 168.4673)
  line L55 (83.9575, 168.4673) -> (82.5048, 166.8108)
  line L56 (82.5048, 166.8108) -> (81.1257, 165.0925)
  line L57 (81.1257, 165.0925) -> (79.8228, 163.3156)
  line L58 (79.8228, 163.3156) -> (78.5987, 161.4836)
  line L59 (78.5987, 161.4836) -> (77.4557, 159.6)
  line L60 (77.4557, 159.6) -> (76.396, 157.6683)
  line L61 (76.396, 157.6683) -> (75.4215, 155.6922)
  line L62 (75.4215, 155.6922) -> (74.5341, 153.6755)
  line L63 (74.5341, 153.6755) -> (73.7355, 151.622)
  line L64 (73.7355, 151.622) -> (73.0273, 149.5356)
  line L65 (73.0273, 149.5356) -> (72.4107, 147.4204)
  line L66 (72.4107, 147.4204) -> (71.9067, 145.3604)
  line L67 (71.9067, 145.3604) -> (71.9067, 123.3396)
  line L68 (71.9067, 123.3396) -> (72.4107, 121.2796)
  line L69 (72.4107, 121.2796) -> (73.0273, 119.1644)
  line L70 (73.0273, 119.1644) -> (73.7355, 117.078)
  line L71 (73.7355, 117.078) -> (74.5341, 115.0245)
  line L72 (74.5341, 115.0245) -> (75.4215, 113.0078)
  line L73 (75.4215, 113.0078) -> (76.396, 111.0317)
  line L74 (76.396, 111.0317) -> (77.4557, 109.1)
  line L75 (77.4557, 109.1) -> (78.5987, 107.2164)
  line L76 (78.5987, 107.2164) -> (79.8228, 105.3844)
  line L77 (79.8228, 105.3844) -> (81.1257, 103.6075)
  line L78 (81.1257, 103.6075) -> (82.5048, 101.8892)
  line L79 (82.5048, 101.8892) -> (83.9575, 100.2327)
  line L80 (83.9575, 100.2327) -> (85.4811, 98.6411)
  line L81 (85.4811, 98.6411) -> (87.0727, 97.1175)
  line L82 (87.0727, 97.1175) -> (88.7292, 95.6648)
  line L83 (88.7292, 95.6648) -> (90.4475, 94.2857)
  line L84 (90.4475, 94.2857) -> (92.2244, 92.9828)
  line L85 (92.2244, 92.9828) -> (94.0564, 91.7587)
  line L86 (94.0564, 91.7587) -> (95.94, 90.6157)
  line L87 (95.94, 90.6157) -> (97.8717, 89.556)
  line L88 (97.8717, 89.556) -> (99.8478, 88.5815)
  line L89 (99.8478, 88.5815) -> (101.8645, 87.6941)
  line L90 (101.8645, 87.6941) -> (103.918, 86.8955)
  line L91 (103.918, 86.8955) -> (104.8937, 86.5643)
  line L92 (104.8937, 86.5643) -> (137.4863, 86.5643)
  line L93 (137.4863, 86.5643) -> (138.462, 86.8955)
  line L94 (138.462, 86.8955) -> (140.5155, 87.6941)
  line L95 (140.5155, 87.6941) -> (142.5322, 88.5815)
  line L96 (142.5322, 88.5815) -> (144.5083, 89.556)
  line L97 (144.5083, 89.556) -> (146.44, 90.6157)
  line L98 (146.44, 90.6157) -> (148.3236, 91.7587)
  line L99 (148.3236, 91.7587) -> (150.1556, 92.9828)
  line L100 (150.1556, 92.9828) -> (151.9325, 94.2857)
  line L101 (151.9325, 94.2857) -> (153.6508, 95.6648)
  line L102 (153.6508, 95.6648) -> (155.3073, 97.1175)
  line L103 (155.3073, 97.1175) -> (156.8989, 98.6411)
  line L104 (156.8989, 98.6411) -> (158.4225, 100.2327)
  line L105 (158.4225, 100.2327) -> (159.8752, 101.8892)
  line L106 (159.8752, 101.8892) -> (161.2543, 103.6075)
  line L107 (161.2543, 103.6075) -> (162.5572, 105.3844)
  line L108 (162.5572, 105.3844) -> (163.7813, 107.2164)
  line L109 (163.7813, 107.2164) -> (164.9243, 109.1)
  line L110 (164.9243, 109.1) -> (165.984, 111.0317)
  line L111 (165.984, 111.0317) -> (166.9585, 113.0078)
  line L112 (166.9585, 113.0078) -> (167.8459, 115.0245)
  line L113 (167.8459, 115.0245) -> (168.6445, 117.078)
  line L114 (168.6445, 117.078) -> (169.3527, 119.1644)
  line L115 (169.3527, 119.1644) -> (169.9693, 121.2796)
  line L116 (169.9693, 121.2796) -> (170.4929, 123.4198)
  line L117 (170.4929, 123.4198) -> (170.9228, 125.5808)
  line L118 (170.9228, 125.5808) -> (171.258, 127.7584)
  line L119 (171.258, 127.7584) -> (171.4978, 129.9486)
  line L120 (171.4978, 129.9486) -> (171.6419, 132.1472)
  line L121 (171.6419, 132.1472) -> (171.69, 134.35)
extrude "Rear Wafer Pocket - Final Clearance" cut sketch "Rear Wafer Pocket - Final Clearance Sketch" along normal blind 8.1